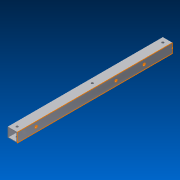
# Autodesk Inventor part: BottomSupportBAse
Saved by Autodesk Inventor 2013 (Build 170138000, 138)
## iProperties
Created: 2013-07-19
Part Number: BottomSupportBAse
Material: Aluminum 6061
Document SubType Name: Modeling
Designer: robotics
Density: 1 g/cm^3
Author: robotics
Autodesk Inventor part; units mm, degrees
ref_plane "YZ Plane" through (0, 0, 0) normal (1, 0, 0) x (0, 1, 0)
ref_plane "XZ Plane" through (0, 0, 0) normal (0, 1, 0) x (-1, 0, 0)
ref_plane "XY Plane" through (0, 0, 0) normal (0, 0, 1) x (1, 0, 0)
sketch "Sketch1" plane through (0, 0, 0) normal (0, 0, 1) x (1, 0, 0)
  line L0 (-10.5156, -10.9728) -> (10.5156, -10.9728)
  line L1 (10.5156, -10.9728) -> (10.5156, 10.9728)
  line L2 (10.5156, 10.9728) -> (-10.5156, 10.9728)
  line L3 (-10.5156, 10.9728) -> (-10.5156, -10.9728)
  line L4 (-10.5156, -10.9728) -> (10.5156, 10.9728) construction
  line L5 (10.5156, -10.9728) -> (-10.5156, 10.9728) construction
  line L6 (-12.7, -12.7) -> (12.7, -12.7)
  line L7 (12.7, -12.7) -> (12.7, 12.7)
  line L8 (12.7, 12.7) -> (-12.7, 12.7)
  line L9 (-12.7, 12.7) -> (-12.7, -12.7)
  line L10 (-12.7, -12.7) -> (12.7, 12.7) construction
  line L11 (12.7, -12.7) -> (-12.7, 12.7) construction
  point P0 (0, 0)
  dimension "d0" = 25.4
  dimension "d2" = 25.4
  dimension "d3" = 1.7272
  dimension "d5" = 2.1844
  constraints: 24 end point, 4 midpoint, 4 parallel, 2 horizontal, 2 perpendicular
  measures "d0" distance of L6.end L7.end
  measures "d2" distance of L6.start L6.end
  measures "d3" distance between parallel lines of L8 L2
  measures "d5" distance between parallel lines of L9 L3
extrude "Extrusion1" add sketch "Sketch1" along normal blind 419.1
sketch "Sketch2" plane through (12.7, -12.7, 0) normal (1, 0, 0) x (0, 0, -1)
  line L0 (0, 0) -> (0, 25.4) projected
  line L1 (0, 25.4) -> (-419.1, 25.4) projected
  line L2 (-419.1, 0) -> (-419.1, 25.4) projected
  point P0 (0, 12.7)
  point P1 (-368.3, 12.7)
  point P2 (-152.4, 12.7)
  point P3 (-76.2, 12.7)
  dimension "d8" = 12.7
  dimension "d9" = 50.8
  dimension "d11" = 76.2
  dimension "d12" = 12.7
  dimension "d13" = 12.7
  dimension "d14" = 76.2
  measures "d8" distance from line of point (-368.3, 12.7) L1
  measures "d9" distance from line of L2 point (-368.3, 12.7)
  measures "d11" distance of point (-76.2, 12.7) point (-152.4, 12.7)
  measures "d12" distance from line of point (-152.4, 12.7) L1
  measures "d13" distance from line of point (-76.2, 12.7) L1
  measures "d14" distance from line of point (-76.2, 12.7) L0
hole "Hole1" at (12.7, 0, 368.3) at (12.7, 0, 152.4) at (12.7, 0, 76.2) direction (-1, 0, 0) diameter 6.35 end through all
sketch "Sketch3" plane through (12.7, -12.7, 0) normal (1, 0, 0) x (0, 0, -1)
  circle A0 centre (-152.4, 12.7) radius 3.175 projected
  circle A1 centre (-368.3, 12.7) radius 3.175 projected
  circle A2 centre (-76.2, 12.7) radius 3.175 projected
  line L0 (0, 0) -> (0, 25.4) projected
  line L1 (0, 25.4) -> (-419.1, 25.4) projected
  line L2 (-419.1, 0) -> (-419.1, 25.4) projected
  line L3 (0, 0) -> (-419.1, 0) projected
  point P0 (0, 12.7)
sketch "Sketch4" plane through (-12.7, -12.7, 0) normal (0, -1, 0) x (1, 0, 0)
  line L0 (0, 0) -> (25.4, 0) projected
  line L1 (25.4, 0) -> (25.4, 419.1) projected
  line L2 (0, 419.1) -> (25.4, 419.1) projected
  line L3 (0, 0) -> (0, 419.1) projected
  point P0 (12.7, 0)
  point P1 (12.7, 406.4)
  point P2 (12.7, 12.7)
  dimension "d22" = 12.7
  dimension "d23" = 12.7
  dimension "d24" = 12.7
  dimension "d25" = 12.7
  measures "d22" distance from line of point (12.7, 406.4) L3
  measures "d23" distance from line of point (12.7, 406.4) L2
  measures "d24" distance from line of L0 point (12.7, 12.7)
  measures "d25" distance from line of L1 point (12.7, 12.7)
hole "Hole2" at (0, -12.7, 12.7) at (0, -12.7, 406.4) direction (0, 1, 0) diameter 6.35 end through all
sketch "Sketch5" plane through (-12.7, -12.7, 0) normal (0, -1, 0) x (1, 0, 0)
  line L0 (0, 0) -> (25.4, 0) projected
  line L1 (25.4, 0) -> (25.4, 419.1) projected
  point P0 (12.7, 0)
  point P1 (12.7, 203.2)
  dimension "d33" = 203.2
  dimension "d34" = 12.7
  measures "d33" distance from line of L0 point (12.7, 203.2)
  measures "d34" distance from line of L1 point (12.7, 203.2)
hole "Hole3" at (0, -12.7, 203.2) direction (0, 1, 0) diameter 6.35 end through all
body "Solid1"
